Autodesk Fusion 360 part; units mm, degrees
(part 4 of 6)
  spline S54 degree 5 poles (54.1906, -36.7461) (54.1649, -36.7627) (54.114, -36.7965) (54.0391, -36.8491) (53.9417, -36.9229) (53.8236, -37.0198) (53.708, -37.1203) (53.594, -37.2229) (53.4808, -37.3266) (53.3682, -37.4312) (53.2562, -37.5365) (53.145, -37.6429) (53.0349, -37.7507) (52.9261, -37.8602) (52.8187, -37.9713) (52.7124, -38.0839) (52.6071, -38.1978) (52.5028, -38.3128) (52.3992, -38.4286) (52.2963, -38.5454) (52.1942, -38.6629) (52.0928, -38.7814) (51.9923, -38.9009) (51.8926, -39.0213) (51.7938, -39.1427) (51.6958, -39.265) (51.5985, -39.3882) (51.502, -39.5122) (51.4062, -39.637) (51.3111, -39.7625) (51.2167, -39.8889) (51.123, -40.0159) (51.03, -40.1437) (50.9377, -40.2723) (50.8462, -40.4016) (50.7553, -40.5316) (50.6651, -40.6624) (50.5755, -40.7938) (50.4867, -40.9259) (50.3985, -41.0586) (50.3109, -41.192) (50.224, -41.3261) (50.1377, -41.4608) (50.0521, -41.5961) (49.9671, -41.7321) (49.8828, -41.8686) (49.7991, -42.0058) (49.716, -42.1435) (49.6335, -42.2819) (49.5517, -42.4208) (49.4705, -42.5603) (49.3899, -42.7004) (49.3099, -42.841) (49.2305, -42.9822) (49.1517, -43.124) (49.0736, -43.2662) (48.996, -43.4091) (48.919, -43.5524) (48.8427, -43.6963) (48.7669, -43.8407) (48.6917, -43.9856) (48.6171, -44.131) (48.5431, -44.2769) (48.4697, -44.4233) (48.3969, -44.5702) (48.3246, -44.7176) (48.253, -44.8654) (48.1819, -45.0138) (48.1114, -45.1626) (48.0414, -45.3118) (47.9721, -45.4616) (47.9171, -45.5817) (47.876, -45.6721) (47.8488, -45.7324) (47.8352, -45.7626) knots 0 0 0 0 0 0 0.01428571 0.02857143 0.04285714 0.05714286 0.07142857 0.08571429 0.1 0.11428571 0.12857143 0.14285714 0.15714286 0.17142857 0.18571429 0.2 0.21428571 0.22857143 0.24285714 0.25714286 0.27142857 0.28571429 0.3 0.31428571 0.32857143 0.34285714 0.35714286 0.37142857 0.38571429 0.4 0.41428571 0.42857143 0.44285714 0.45714286 0.47142857 0.48571429 0.5 0.51428571 0.52857143 0.54285714 0.55714286 0.57142857 0.58571429 0.6 0.61428571 0.62857143 0.64285714 0.65714286 0.67142857 0.68571429 0.7 0.71428571 0.72857143 0.74285714 0.75714286 0.77142857 0.78571429 0.8 0.81428571 0.82857143 0.84285714 0.85714286 0.87142857 0.88571429 0.9 0.91428571 0.92857143 0.94285714 0.95714286 0.97142857 0.98571429 1 1 1 1 1 1
  arc A111 (47.8352, -45.7626) -> (50.4485, -49.1682) centre (111, 0) ccw
  spline S55 degree 5 poles (50.4485, -49.1682) (50.4812, -49.1629) (50.5465, -49.1523) (50.6443, -49.136) (50.7747, -49.114) (50.9372, -49.0857) (51.0995, -49.0568) (51.2615, -49.0272) (51.4232, -48.997) (51.5846, -48.966) (51.7456, -48.9344) (51.9064, -48.902) (52.0668, -48.869) (52.2269, -48.8353) (52.3866, -48.8009) (52.5461, -48.7658) (52.7051, -48.73) (52.8639, -48.6934) (53.0222, -48.6562) (53.1803, -48.6182) (53.3379, -48.5795) (53.4952, -48.5401) (53.6522, -48.5) (53.8087, -48.4591) (53.9649, -48.4175) (54.1206, -48.3752) (54.276, -48.3321) (54.431, -48.2883) (54.5856, -48.2437) (54.7397, -48.1983) (54.8935, -48.1522) (55.0468, -48.1053) (55.1996, -48.0576) (55.3521, -48.0091) (55.504, -47.9599) (55.6556, -47.9098) (55.8066, -47.859) (55.9572, -47.8073) (56.1073, -47.7549) (56.257, -47.7016) (56.4061, -47.6474) (56.5547, -47.5924) (56.7028, -47.5366) (56.8503, -47.4799) (56.9973, -47.4222) (57.1437, -47.3638) (57.2896, -47.3044) (57.4349, -47.2442) (57.5797, -47.183) (57.7238, -47.121) (57.8674, -47.0579) (58.0102, -46.9939) (58.1523, -46.9288) (58.2937, -46.8626) (58.4344, -46.7954) (58.5744, -46.7271) (58.7138, -46.658) (58.8525, -46.5879) (58.9906, -46.5169) (59.1278, -46.4447) (59.2641, -46.3712) (59.3992, -46.2961) (59.5331, -46.2194) (59.6658, -46.141) (59.7973, -46.0611) (59.928, -45.9802) (60.0582, -45.8985) (60.1877, -45.816) (60.3163, -45.7324) (60.4433, -45.6467) (60.5675, -45.5577) (60.6639, -45.4828) (60.7341, -45.424) (60.7799, -45.3836) (60.8026, -45.3631) knots -1 -1 -1 -1 -1 -1 -0.98571429 -0.97142857 -0.95714286 -0.94285714 -0.92857143 -0.91428571 -0.9 -0.88571429 -0.87142857 -0.85714286 -0.84285714 -0.82857143 -0.81428571 -0.8 -0.78571429 -0.77142857 -0.75714286 -0.74285714 -0.72857143 -0.71428571 -0.7 -0.68571429 -0.67142857 -0.65714286 -0.64285714 -0.62857143 -0.61428571 -0.6 -0.58571429 -0.57142857 -0.55714286 -0.54285714 -0.52857143 -0.51428571 -0.5 -0.48571429 -0.47142857 -0.45714286 -0.44285714 -0.42857143 -0.41428571 -0.4 -0.38571429 -0.37142857 -0.35714286 -0.34285714 -0.32857143 -0.31428571 -0.3 -0.28571429 -0.27142857 -0.25714286 -0.24285714 -0.22857143 -0.21428571 -0.2 -0.18571429 -0.17142857 -0.15714286 -0.14285714 -0.12857143 -0.11428571 -0.1 -0.08571429 -0.07142857 -0.05714286 -0.04285714 -0.02857143 -0.01428571 0 0 0 0 0 0
  line L55 (60.8026, -45.3631) -> (61.2698, -44.9409)
  arc A112 (64.054, -45.0401) -> (61.2698, -44.9409) centre (62.6108, -46.4248) ccw
  arc A113 (64.054, -45.0401) -> (65.9599, -46.946) centre (111, 0) ccw
  arc A114 (66.0591, -49.7302) -> (65.9599, -46.946) centre (64.5752, -48.3892) ccw
  line L56 (66.0591, -49.7302) -> (65.6369, -50.1974)
  spline S56 degree 5 poles (65.6369, -50.1974) (65.6164, -50.2201) (65.576, -50.2659) (65.5172, -50.3361) (65.4423, -50.4325) (65.3533, -50.5567) (65.2676, -50.6837) (65.184, -50.8123) (65.1015, -50.9418) (65.0198, -51.072) (64.9389, -51.2027) (64.859, -51.3342) (64.7806, -51.4669) (64.7039, -51.6008) (64.6288, -51.7359) (64.5553, -51.8722) (64.4831, -52.0094) (64.4121, -52.1475) (64.342, -52.2862) (64.2729, -52.4256) (64.2046, -52.5656) (64.1374, -52.7063) (64.0712, -52.8477) (64.0061, -52.9898) (63.9421, -53.1326) (63.879, -53.2762) (63.817, -53.4203) (63.7558, -53.5651) (63.6956, -53.7104) (63.6362, -53.8563) (63.5778, -54.0027) (63.5201, -54.1497) (63.4634, -54.2972) (63.4076, -54.4453) (63.3526, -54.5939) (63.2984, -54.743) (63.2451, -54.8927) (63.1927, -55.0428) (63.141, -55.1934) (63.0902, -55.3444) (63.0401, -55.496) (62.9909, -55.6479) (62.9424, -55.8004) (62.8947, -55.9532) (62.8478, -56.1065) (62.8017, -56.2603) (62.7563, -56.4144) (62.7117, -56.569) (62.6679, -56.724) (62.6248, -56.8794) (62.5825, -57.0351) (62.5409, -57.1913) (62.5, -57.3478) (62.4599, -57.5048) (62.4205, -57.6621) (62.3818, -57.8197) (62.3438, -57.9778) (62.3066, -58.1361) (62.27, -58.2949) (62.2342, -58.4539) (62.1991, -58.6134) (62.1647, -58.7731) (62.131, -58.9332) (62.098, -59.0936) (62.0656, -59.2544) (62.034, -59.4154) (62.003, -59.5768) (61.9728, -59.7385) (61.9432, -59.9005) (61.9143, -60.0628) (61.886, -60.2253) (61.864, -60.3557) (61.8477, -60.4535) (61.8371, -60.5188) (61.8318, -60.5515) knots 0 0 0 0 0 0 0.01428571 0.02857143 0.04285714 0.05714286 0.07142857 0.08571429 0.1 0.11428571 0.12857143 0.14285714 0.15714286 0.17142857 0.18571429 0.2 0.21428571 0.22857143 0.24285714 0.25714286 0.27142857 0.28571429 0.3 0.31428571 0.32857143 0.34285714 0.35714286 0.37142857 0.38571429 0.4 0.41428571 0.42857143 0.44285714 0.45714286 0.47142857 0.48571429 0.5 0.51428571 0.52857143 0.54285714 0.55714286 0.57142857 0.58571429 0.6 0.61428571 0.62857143 0.64285714 0.65714286 0.67142857 0.68571429 0.7 0.71428571 0.72857143 0.74285714 0.75714286 0.77142857 0.78571429 0.8 0.81428571 0.82857143 0.84285714 0.85714286 0.87142857 0.88571429 0.9 0.91428571 0.92857143 0.94285714 0.95714286 0.97142857 0.98571429 1 1 1 1 1 1
  arc A115 (61.8318, -60.5515) -> (65.2374, -63.1648) centre (111, 0) ccw
  spline S57 degree 5 poles (65.2374, -63.1648) (65.2676, -63.1512) (65.3279, -63.124) (65.4183, -63.0829) (65.5384, -63.0279) (65.6882, -62.9586) (65.8374, -62.8886) (65.9862, -62.8181) (66.1346, -62.747) (66.2824, -62.6754) (66.4298, -62.6031) (66.5767, -62.5303) (66.7231, -62.4569) (66.869, -62.3829) (67.0144, -62.3083) (67.1593, -62.2331) (67.3037, -62.1573) (67.4476, -62.081) (67.5909, -62.004) (67.7338, -61.9264) (67.876, -61.8483) (68.0178, -61.7695) (68.159, -61.6901) (68.2996, -61.6101) (68.4397, -61.5295) (68.5792, -61.4483) (68.7181, -61.3665) (68.8565, -61.284) (68.9942, -61.2009) (69.1314, -61.1172) (69.2679, -61.0329) (69.4039, -60.9479) (69.5392, -60.8623) (69.6739, -60.776) (69.808, -60.6891) (69.9414, -60.6015) (70.0741, -60.5133) (70.2062, -60.4245) (70.3376, -60.3349) (70.4684, -60.2447) (70.5984, -60.1538) (70.7277, -60.0623) (70.8563, -59.97) (70.9841, -59.877) (71.1111, -59.7833) (71.2375, -59.6889) (71.363, -59.5938) (71.4878, -59.498) (71.6118, -59.4015) (71.735, -59.3042) (71.8573, -59.2062) (71.9787, -59.1074) (72.0991, -59.0077) (72.2186, -58.9072) (72.3371, -58.8058) (72.4546, -58.7037) (72.5714, -58.6008) (72.6872, -58.4972) (72.8022, -58.3929) (72.9161, -58.2876) (73.0287, -58.1813) (73.1398, -58.0739) (73.2493, -57.9651) (73.3571, -57.855) (73.4635, -57.7438) (73.5688, -57.6318) (73.6734, -57.5192) (73.7771, -57.406) (73.8797, -57.292) (73.9802, -57.1764) (74.0771, -57.0583) (74.1509, -56.9609) (74.2035, -56.886) (74.2373, -56.8351) (74.2539, -56.8094) knots -1 -1 -1 -1 -1 -1 -0.98571429 -0.97142857 -0.95714286 -0.94285714 -0.92857143 -0.91428571 -0.9 -0.88571429 -0.87142857 -0.85714286 -0.84285714 -0.82857143 -0.81428571 -0.8 -0.78571429 -0.77142857 -0.75714286 -0.74285714 -0.72857143 -0.71428571 -0.7 -0.68571429 -0.67142857 -0.65714286 -0.64285714 -0.62857143 -0.61428571 -0.6 -0.58571429 -0.57142857 -0.55714286 -0.54285714 -0.52857143 -0.51428571 -0.5 -0.48571429 -0.47142857 -0.45714286 -0.44285714 -0.42857143 -0.41428571 -0.4 -0.38571429 -0.37142857 -0.35714286 -0.34285714 -0.32857143 -0.31428571 -0.3 -0.28571429 -0.27142857 -0.25714286 -0.24285714 -0.22857143 -0.21428571 -0.2 -0.18571429 -0.17142857 -0.15714286 -0.14285714 -0.12857143 -0.11428571 -0.1 -0.08571429 -0.07142857 -0.05714286 -0.04285714 -0.02857143 -0.01428571 0 0 0 0 0 0
  line L57 (74.2539, -56.8094) -> (74.5959, -56.2807)
  arc A116 (77.3109, -55.656) -> (74.5959, -56.2807) centre (76.2752, -57.3669) ccw
  arc A117 (77.3109, -55.656) -> (79.6451, -57.0036) centre (111, 0) ccw
  arc A118 (80.4615, -59.6672) -> (79.6451, -57.0036) centre (78.6812, -58.756) ccw
  line L58 (80.4615, -59.6672) -> (80.1746, -60.2278)
  spline S58 degree 5 poles (80.1746, -60.2278) (80.1607, -60.255) (80.1336, -60.3097) (80.095, -60.3928) (80.0475, -60.5053) (79.9937, -60.6483) (79.9438, -60.7931) (79.8964, -60.939) (79.8502, -61.0854) (79.8049, -61.2323) (79.7606, -61.3795) (79.7175, -61.5272) (79.6761, -61.6756) (79.6367, -61.8248) (79.5991, -61.9748) (79.5634, -62.1255) (79.5292, -62.2767) (79.4963, -62.4284) (79.4645, -62.5806) (79.4338, -62.7331) (79.4041, -62.886) (79.3756, -63.0393) (79.3483, -63.193) (79.3222, -63.3471) (79.2973, -63.5017) (79.2735, -63.6566) (79.2509, -63.8119) (79.2293, -63.9676) (79.2087, -64.1236) (79.1892, -64.2798) (79.1706, -64.4364) (79.153, -64.5933) (79.1363, -64.7505) (79.1207, -64.908) (79.1061, -65.0657) (79.0924, -65.2238) (79.0796, -65.3821) (79.0678, -65.5407) (79.0569, -65.6995) (79.0468, -65.8586) (79.0377, -66.0179) (79.0295, -66.1775) (79.0221, -66.3372) (79.0156, -66.4972) (79.01, -66.6575) (79.0052, -66.8179) (79.0013, -66.9785) (78.9983, -67.1394) (78.996, -67.3004) (78.9946, -67.4617) (78.994, -67.6231) (78.9943, -67.7847) (78.9953, -67.9465) (78.9972, -68.1085) (78.9998, -68.2706) (79.0033, -68.4329) (79.0075, -68.5954) (79.0125, -68.758) (79.0183, -68.9208) (79.0249, -69.0837) (79.0322, -69.2468) (79.0403, -69.41) (79.0492, -69.5733) (79.0588, -69.7368) (79.0692, -69.9005) (79.0803, -70.0642) (79.0922, -70.2281) (79.1048, -70.3921) (79.1181, -70.5563) (79.1322, -70.7205) (79.147, -70.8848) (79.1594, -71.0164) (79.1691, -71.1152) (79.1757, -71.181) (79.179, -71.2139) knots 0 0 0 0 0 0 0.01428571 0.02857143 0.04285714 0.05714286 0.07142857 0.08571429 0.1 0.11428571 0.12857143 0.14285714 0.15714286 0.17142857 0.18571429 0.2 0.21428571 0.22857143 0.24285714 0.25714286 0.27142857 0.28571429 0.3 0.31428571 0.32857143 0.34285714 0.35714286 0.37142857 0.38571429 0.4 0.41428571 0.42857143 0.44285714 0.45714286 0.47142857 0.48571429 0.5 0.51428571 0.52857143 0.54285714 0.55714286 0.57142857 0.58571429 0.6 0.61428571 0.62857143 0.64285714 0.65714286 0.67142857 0.68571429 0.7 0.71428571 0.72857143 0.74285714 0.75714286 0.77142857 0.78571429 0.8 0.81428571 0.82857143 0.84285714 0.85714286 0.87142857 0.88571429 0.9 0.91428571 0.92857143 0.94285714 0.95714286 0.97142857 0.98571429 1 1 1 1 1 1
  arc A119 (79.179, -71.2139) -> (83.145, -72.8567) centre (111, 0) ccw
  spline S59 degree 5 poles (83.145, -72.8567) (83.1706, -72.8358) (83.2218, -72.7939) (83.2985, -72.7309) (83.4003, -72.6466) (83.527, -72.5409) (83.6531, -72.4347) (83.7786, -72.3281) (83.9035, -72.221) (84.0277, -72.1135) (84.1514, -72.0056) (84.2744, -71.8972) (84.3969, -71.7884) (84.5186, -71.6792) (84.6398, -71.5695) (84.7603, -71.4594) (84.8801, -71.3488) (84.9993, -71.2378) (85.1179, -71.1264) (85.2358, -71.0145) (85.353, -70.9021) (85.4695, -70.7894) (85.5853, -70.6762) (85.7004, -70.5625) (85.8149, -70.4484) (85.9286, -70.3338) (86.0416, -70.2188) (86.1539, -70.1034) (86.2655, -69.9875) (86.3763, -69.8711) (86.4864, -69.7543) (86.5957, -69.637) (86.7043, -69.5193) (86.8121, -69.4011) (86.919, -69.2825) (87.0252, -69.1634) (87.1306, -69.0438) (87.2352, -68.9238) (87.339, -68.8033) (87.4419, -68.6823) (87.544, -68.5608) (87.6452, -68.4389) (87.7455, -68.3165) (87.8449, -68.1936) (87.9434, -68.0702) (88.041, -67.9464) (88.1376, -67.822) (88.2334, -67.6972) (88.3282, -67.5719) (88.422, -67.446) (88.5147, -67.3197) (88.6064, -67.1928) (88.6969, -67.0653) (88.7863, -66.9373) (88.8745, -66.8088) (88.9617, -66.6797) (89.0478, -66.5501) (89.1329, -66.4201) (89.2169, -66.2895) (89.2997, -66.1584) (89.381, -66.0266) (89.4605, -65.894) (89.5381, -65.7606) (89.6137, -65.6264) (89.6877, -65.4914) (89.7605, -65.356) (89.8323, -65.2202) (89.9032, -65.084) (89.9728, -64.9473) (90.0399, -64.8096) (90.103, -64.6704) (90.149, -64.5573) (90.1805, -64.4713) (90.2, -64.4134) (90.2094, -64.3843) knots -1 -1 -1 -1 -1 -1 -0.98571429 -0.97142857 -0.95714286 -0.94285714 -0.92857143 -0.91428571 -0.9 -0.88571429 -0.87142857 -0.85714286 -0.84285714 -0.82857143 -0.81428571 -0.8 -0.78571429 -0.77142857 -0.75714286 -0.74285714 -0.72857143 -0.71428571 -0.7 -0.68571429 -0.67142857 -0.65714286 -0.64285714 -0.62857143 -0.61428571 -0.6 -0.58571429 -0.57142857 -0.55714286 -0.54285714 -0.52857143 -0.51428571 -0.5 -0.48571429 -0.47142857 -0.45714286 -0.44285714 -0.42857143 -0.41428571 -0.4 -0.38571429 -0.37142857 -0.35714286 -0.34285714 -0.32857143 -0.31428571 -0.3 -0.28571429 -0.27142857 -0.25714286 -0.24285714 -0.22857143 -0.21428571 -0.2 -0.18571429 -0.17142857 -0.15714286 -0.14285714 -0.12857143 -0.11428571 -0.1 -0.08571429 -0.07142857 -0.05714286 -0.04285714 -0.02857143 -0.01428571 0 0 0 0 0 0
  line L59 (90.2094, -64.3843) -> (90.4029, -63.7851)
  arc A120 (92.8636, -62.4789) -> (90.4029, -63.7851) centre (92.3061, -64.3996) ccw
  arc A121 (92.8636, -62.4789) -> (95.4671, -63.1765) centre (111, 0) ccw
  arc A122 (96.9451, -65.538) -> (95.4671, -63.1765) centre (94.9896, -65.1187) ccw
  line L60 (96.9451, -65.538) -> (96.8131, -66.1537)
  spline S60 degree 5 poles (96.8131, -66.1537) (96.8067, -66.1836) (96.7946, -66.2435) (96.7788, -66.3338) (96.7621, -66.4547) (96.7471, -66.6068) (96.7364, -66.7596) (96.7284, -66.9128) (96.7217, -67.0662) (96.716, -67.2197) (96.7113, -67.3734) (96.7079, -67.5272) (96.7063, -67.6813) (96.7068, -67.8356) (96.7093, -67.9902) (96.7138, -68.145) (96.7199, -68.2999) (96.7274, -68.455) (96.7361, -68.6102) (96.7459, -68.7655) (96.7568, -68.9208) (96.769, -69.0763) (96.7823, -69.2318) (96.797, -69.3875) (96.813, -69.5432) (96.8301, -69.699) (96.8485, -69.8549) (96.8679, -70.0108) (96.8884, -70.1668) (96.9099, -70.3228) (96.9325, -70.4789) (96.9561, -70.635) (96.9807, -70.7911) (97.0064, -70.9473) (97.0331, -71.1034) (97.0607, -71.2596) (97.0894, -71.4159) (97.119, -71.5721) (97.1496, -71.7284) (97.1811, -71.8846) (97.2135, -72.0409) (97.2468, -72.1971) (97.2811, -72.3533) (97.3162, -72.5096) (97.3523, -72.6658) (97.3892, -72.822) (97.427, -72.9782) (97.4656, -73.1343) (97.5052, -73.2905) (97.5455, -73.4466) (97.5868, -73.6026) (97.6288, -73.7587) (97.6717, -73.9147) (97.7154, -74.0707) (97.7599, -74.2266) (97.8053, -74.3825) (97.8514, -74.5383) (97.8983, -74.6941) (97.9461, -74.8498) (97.9946, -75.0055) (98.0439, -75.1611) (98.0939, -75.3167) (98.1448, -75.4722) (98.1964, -75.6276) (98.2488, -75.783) (98.3019, -75.9383) (98.3558, -76.0935) (98.4104, -76.2487) (98.4658, -76.4037) (98.5219, -76.5587) (98.5787, -76.7137) (98.6248, -76.8375) (98.6597, -76.9304) (98.6831, -76.9923) (98.6948, -77.0233) knots 0 0 0 0 0 0 0.01428571 0.02857143 0.04285714 0.05714286 0.07142857 0.08571429 0.1 0.11428571 0.12857143 0.14285714 0.15714286 0.17142857 0.18571429 0.2 0.21428571 0.22857143 0.24285714 0.25714286 0.27142857 0.28571429 0.3 0.31428571 0.32857143 0.34285714 0.35714286 0.37142857 0.38571429 0.4 0.41428571 0.42857143 0.44285714 0.45714286 0.47142857 0.48571429 0.5 0.51428571 0.52857143 0.54285714 0.55714286 0.57142857 0.58571429 0.6 0.61428571 0.62857143 0.64285714 0.65714286 0.67142857 0.68571429 0.7 0.71428571 0.72857143 0.74285714 0.75714286 0.77142857 0.78571429 0.8 0.81428571 0.82857143 0.84285714 0.85714286 0.87142857 0.88571429 0.9 0.91428571 0.92857143 0.94285714 0.95714286 0.97142857 0.98571429 1 1 1 1 1 1
  arc A123 (98.6948, -77.0233) -> (102.9508, -77.5836) centre (111, 0) ccw
  spline S61 degree 5 poles (102.9508, -77.5836) (102.9702, -77.5567) (103.0088, -77.503) (103.0665, -77.4223) (103.1431, -77.3146) (103.2381, -77.1796) (103.3324, -77.0444) (103.426, -76.909) (103.5189, -76.7732) (103.6111, -76.6373) (103.7027, -76.501) (103.7935, -76.3645) (103.8835, -76.2277) (103.9729, -76.0906) (104.0615, -75.9533) (104.1494, -75.8158) (104.2366, -75.678) (104.323, -75.5399) (104.4087, -75.4016) (104.4935, -75.263) (104.5777, -75.1242) (104.661, -74.9851) (104.7436, -74.8457) (104.8254, -74.7061) (104.9064, -74.5663) (104.9866, -74.4262) (105.066, -74.2859) (105.1446, -74.1453) (105.2224, -74.0045) (105.2993, -73.8634) (105.3754, -73.7221) (105.4507, -73.5805) (105.5251, -73.4387) (105.5986, -73.2966) (105.6712, -73.1543) (105.743, -73.0118) (105.8138, -72.869) (105.8838, -72.726) (105.9528, -72.5828) (106.0209, -72.4393) (106.0881, -72.2956) (106.1543, -72.1516) (106.2195, -72.0074) (106.2837, -71.863) (106.3469, -71.7183) (106.4091, -71.5734) (106.4703, -71.4283) (106.5304, -71.2829) (106.5896, -71.1373) (106.6476, -70.9915) (106.7045, -70.8454) (106.7602, -70.6991) (106.8147, -70.5526) (106.8679, -70.4058) (106.9198, -70.2588) (106.9706, -70.1116) (107.0202, -69.9641) (107.0688, -69.8165) (107.1162, -69.6686) (107.1622, -69.5205) (107.2066, -69.3722) (107.249, -69.2235) (107.2894, -69.0746) (107.3278, -68.9254) (107.3644, -68.7759) (107.3996, -68.6262) (107.4338, -68.4764) (107.467, -68.3265) (107.4989, -68.1765) (107.5281, -68.0261) (107.553, -67.8753) (107.5682, -67.7542) (107.5763, -67.663) (107.5801, -67.602) (107.5817, -67.5715) knots -1 -1 -1 -1 -1 -1 -0.98571429 -0.97142857 -0.95714286 -0.94285714 -0.92857143 -0.91428571 -0.9 -0.88571429 -0.87142857 -0.85714286 -0.84285714 -0.82857143 -0.81428571 -0.8 -0.78571429 -0.77142857 -0.75714286 -0.74285714 -0.72857143 -0.71428571 -0.7 -0.68571429 -0.67142857 -0.65714286 -0.64285714 -0.62857143 -0.61428571 -0.6 -0.58571429 -0.57142857 -0.55714286 -0.54285714 -0.52857143 -0.51428571 -0.5 -0.48571429 -0.47142857 -0.45714286 -0.44285714 -0.42857143 -0.41428571 -0.4 -0.38571429 -0.37142857 -0.35714286 -0.34285714 -0.32857143 -0.31428571 -0.3 -0.28571429 -0.27142857 -0.25714286 -0.24285714 -0.22857143 -0.21428571 -0.2 -0.18571429 -0.17142857 -0.15714286 -0.14285714 -0.12857143 -0.11428571 -0.1 -0.08571429 -0.07142857 -0.05714286 -0.04285714 -0.02857143 -0.01428571 0 0 0 0 0 0
  line L61 (107.5817, -67.5715) -> (107.6135, -66.9426)
  arc A124 (109.6523, -65.044) -> (107.6135, -66.9426) centre (109.6109, -67.0436) ccw
  arc A125 (109.6523, -65.044) -> (112.3477, -65.044) centre (111, 0) ccw
  arc A126 (114.3865, -66.9426) -> (112.3477, -65.044) centre (112.3891, -67.0436) ccw
  line L62 (114.3865, -66.9426) -> (114.4183, -67.5715)
  spline S62 degree 5 poles (114.4183, -67.5715) (114.4199, -67.602) (114.4237, -67.663) (114.4318, -67.7542) (114.447, -67.8753) (114.4719, -68.0261) (114.5011, -68.1765) (114.533, -68.3265) (114.5662, -68.4764) (114.6004, -68.6262) (114.6356, -68.7759) (114.6722, -68.9254) (114.7106, -69.0746) (114.751, -69.2235) (114.7934, -69.3722) (114.8378, -69.5205) (114.8838, -69.6686) (114.9312, -69.8165) (114.9798, -69.9641) (115.0294, -70.1116) (115.0802, -70.2588) (115.1321, -70.4058) (115.1853, -70.5526) (115.2398, -70.6991) (115.2955, -70.8454) (115.3524, -70.9915) (115.4104, -71.1373) (115.4696, -71.2829) (115.5297, -71.4283) (115.5909, -71.5734) (115.6531, -71.7183) (115.7163, -71.863) (115.7805, -72.0074) (115.8457, -72.1516) (115.9119, -72.2956) (115.9791, -72.4393) (116.0472, -72.5828) (116.1162, -72.726) (116.1862, -72.869) (116.257, -73.0118) (116.3288, -73.1543) (116.4014, -73.2966) (116.4749, -73.4387) (116.5493, -73.5805) (116.6246, -73.7221) (116.7007, -73.8634) (116.7776, -74.0045) (116.8554, -74.1453) (116.934, -74.2859) (117.0134, -74.4262) (117.0936, -74.5663) (117.1746, -74.7061) (117.2564, -74.8457) (117.339, -74.9851) (117.4223, -75.1242) (117.5065, -75.263) (117.5913, -75.4016) (117.677, -75.5399) (117.7634, -75.678) (117.8506, -75.8158) (117.9385, -75.9533) (118.0271, -76.0906) (118.1165, -76.2277) (118.2065, -76.3645) (118.2973, -76.501) (118.3889, -76.6373) (118.4811, -76.7732) (118.574, -76.909) (118.6676, -77.0444) (118.7619, -77.1796) (118.8569, -77.3146) (118.9335, -77.4223) (118.9912, -77.503) (119.0298, -77.5567) (119.0492, -77.5836) knots 0 0 0 0 0 0 0.01428571 0.02857143 0.04285714 0.05714286 0.07142857 0.08571429 0.1 0.11428571 0.12857143 0.14285714 0.15714286 0.17142857 0.18571429 0.2 0.21428571 0.22857143 0.24285714 0.25714286 0.27142857 0.28571429 0.3 0.31428571 0.32857143 0.34285714 0.35714286 0.37142857 0.38571429 0.4 0.41428571 0.42857143 0.44285714 0.45714286 0.47142857 0.48571429 0.5 0.51428571 0.52857143 0.54285714 0.55714286 0.57142857 0.58571429 0.6 0.61428571 0.62857143 0.64285714 0.65714286 0.67142857 0.68571429 0.7 0.71428571 0.72857143 0.74285714 0.75714286 0.77142857 0.78571429 0.8 0.81428571 0.82857143 0.84285714 0.85714286 0.87142857 0.88571429 0.9 0.91428571 0.92857143 0.94285714 0.95714286 0.97142857 0.98571429 1 1 1 1 1 1
  arc A127 (119.0492, -77.5836) -> (123.3052, -77.0233) centre (111, 0) ccw
  spline S63 degree 5 poles (123.3052, -77.0233) (123.3169, -76.9923) (123.3403, -76.9304) (123.3752, -76.8375) (123.4213, -76.7137) (123.4781, -76.5587) (123.5342, -76.4037) (123.5896, -76.2487) (123.6442, -76.0935) (123.6981, -75.9383) (123.7512, -75.783) (123.8036, -75.6276) (123.8552, -75.4722) (123.9061, -75.3167) (123.9561, -75.1611) (124.0054, -75.0055) (124.0539, -74.8498) (124.1017, -74.6941) (124.1486, -74.5383) (124.1947, -74.3825) (124.2401, -74.2266) (124.2846, -74.0707) (124.3283, -73.9147) (124.3712, -73.7587) (124.4132, -73.6026) (124.4545, -73.4466) (124.4948, -73.2905) (124.5344, -73.1343) (124.573, -72.9782) (124.6108, -72.822) (124.6477, -72.6658) (124.6838, -72.5096) (124.7189, -72.3533) (124.7532, -72.1971) (124.7865, -72.0409) (124.8189, -71.8846) (124.8504, -71.7284) (124.881, -71.5721) (124.9106, -71.4159) (124.9393, -71.2596) (124.9669, -71.1034) (124.9936, -70.9473) (125.0193, -70.7911) (125.0439, -70.635) (125.0675, -70.4789) (125.0901, -70.3228) (125.1116, -70.1668) (125.1321, -70.0108) (125.1515, -69.8549) (125.1699, -69.699) (125.187, -69.5432) (125.203, -69.3875) (125.2177, -69.2318) (125.231, -69.0763) (125.2432, -68.9208) (125.2541, -68.7655) (125.2639, -68.6102) (125.2726, -68.455) (125.2801, -68.2999) (125.2862, -68.145) (125.2907, -67.9902) (125.2932, -67.8356) (125.2937, -67.6813) (125.2921, -67.5272) (125.2887, -67.3734) (125.284, -67.2197) (125.2783, -67.0662) (125.2716, -66.9128) (125.2636, -66.7596) (125.2529, -66.6068) (125.2379, -66.4547) (125.2212, -66.3338) (125.2054, -66.2435) (125.1933, -66.1836) (125.1869, -66.1537) knots -1 -1 -1 -1 -1 -1 -0.98571429 -0.97142857 -0.95714286 -0.94285714 -0.92857143 -0.91428571 -0.9 -0.88571429 -0.87142857 -0.85714286 -0.84285714 -0.82857143 -0.81428571 -0.8 -0.78571429 -0.77142857 -0.75714286 -0.74285714 -0.72857143 -0.71428571 -0.7 -0.68571429 -0.67142857 -0.65714286 -0.64285714 -0.62857143 -0.61428571 -0.6 -0.58571429 -0.57142857 -0.55714286 -0.54285714 -0.52857143 -0.51428571 -0.5 -0.48571429 -0.47142857 -0.45714286 -0.44285714 -0.42857143 -0.41428571 -0.4 -0.38571429 -0.37142857 -0.35714286 -0.34285714 -0.32857143 -0.31428571 -0.3 -0.28571429 -0.27142857 -0.25714286 -0.24285714 -0.22857143 -0.21428571 -0.2 -0.18571429 -0.17142857 -0.15714286 -0.14285714 -0.12857143 -0.11428571 -0.1 -0.08571429 -0.07142857 -0.05714286 -0.04285714 -0.02857143 -0.01428571 0 0 0 0 0 0
  line L63 (125.1869, -66.1537) -> (125.0549, -65.538)
  arc A128 (126.5329, -63.1765) -> (125.0549, -65.538) centre (127.0104, -65.1187) ccw
  arc A129 (126.5329, -63.1765) -> (129.1364, -62.4789) centre (111, 0) ccw
  arc A130 (131.5971, -63.7851) -> (129.1364, -62.4789) centre (129.6939, -64.3996) ccw
  line L64 (131.5971, -63.7851) -> (131.7906, -64.3843)
  spline S64 degree 5 poles (131.7906, -64.3843) (131.8, -64.4134) (131.8195, -64.4713) (131.851, -64.5573) (131.897, -64.6704) (131.9601, -64.8096) (132.0272, -64.9473) (132.0968, -65.084) (132.1677, -65.2202) (132.2395, -65.356) (132.3123, -65.4914) (132.3863, -65.6264) (132.4619, -65.7606) (132.5395, -65.894) (132.619, -66.0266) (132.7003, -66.1584) (132.7831, -66.2895) (132.8671, -66.4201) (132.9522, -66.5501) (133.0383, -66.6797) (133.1255, -66.8088) (133.2137, -66.9373) (133.3031, -67.0653) (133.3936, -67.1928) (133.4853, -67.3197) (133.578, -67.446) (133.6718, -67.5719) (133.7666, -67.6972) (133.8624, -67.822) (133.959, -67.9464) (134.0566, -68.0702) (134.1551, -68.1936) (134.2545, -68.3165) (134.3548, -68.4389) (134.456, -68.5608) (134.5581, -68.6823) (134.661, -68.8033) (134.7648, -68.9238) (134.8694, -69.0438) (134.9748, -69.1634) (135.081, -69.2825) (135.1879, -69.4011) (135.2957, -69.5193) (135.4043, -69.637) (135.5136, -69.7543) (135.6237, -69.8711) (135.7345, -69.9875) (135.8461, -70.1034) (135.9584, -70.2188) (136.0714, -70.3338) (136.1851, -70.4484) (136.2996, -70.5625) (136.4147, -70.6762) (136.5305, -70.7894) (136.647, -70.9021) (136.7642, -71.0145) (136.8821, -71.1264) (137.0007, -71.2378) (137.1199, -71.3488) (137.2397, -71.4594) (137.3602, -71.5695) (137.4814, -71.6792) (137.6031, -71.7884) (137.7256, -71.8972) (137.8486, -72.0056) (137.9723, -72.1135) (138.0965, -72.221) (138.2214, -72.3281) (138.3469, -72.4347) (138.473, -72.5409) (138.5997, -72.6466) (138.7015, -72.7309) (138.7782, -72.7939) (138.8294, -72.8358) (138.855, -72.8567) knots 0 0 0 0 0 0 0.01428571 0.02857143 0.04285714 0.05714286 0.07142857 0.08571429 0.1 0.11428571 0.12857143 0.14285714 0.15714286 0.17142857 0.18571429 0.2 0.21428571 0.22857143 0.24285714 0.25714286 0.27142857 0.28571429 0.3 0.31428571 0.32857143 0.34285714 0.35714286 0.37142857 0.38571429 0.4 0.41428571 0.42857143 0.44285714 0.45714286 0.47142857 0.48571429 0.5 0.51428571 0.52857143 0.54285714 0.55714286 0.57142857 0.58571429 0.6 0.61428571 0.62857143 0.64285714 0.65714286 0.67142857 0.68571429 0.7 0.71428571 0.72857143 0.74285714 0.75714286 0.77142857 0.78571429 0.8 0.81428571 0.82857143 0.84285714 0.85714286 0.87142857 0.88571429 0.9 0.91428571 0.92857143 0.94285714 0.95714286 0.97142857 0.98571429 1 1 1 1 1 1
  arc A131 (138.855, -72.8567) -> (142.821, -71.2139) centre (111, 0) ccw
  spline S65 degree 5 poles (142.821, -71.2139) (142.8243, -71.181) (142.8309, -71.1152) (142.8406, -71.0164) (142.853, -70.8848) (142.8678, -70.7205) (142.8819, -70.5563) (142.8952, -70.3921) (142.9078, -70.2281) (142.9197, -70.0642) (142.9308, -69.9005) (142.9412, -69.7368) (142.9508, -69.5733) (142.9597, -69.41) (142.9678, -69.2468) (142.9751, -69.0837) (142.9817, -68.9208) (142.9875, -68.758) (142.9925, -68.5954) (142.9967, -68.4329) (143.0002, -68.2706) (143.0028, -68.1085) (143.0047, -67.9465) (143.0057, -67.7847) (143.006, -67.6231) (143.0054, -67.4617) (143.004, -67.3004) (143.0017, -67.1394) (142.9987, -66.9785) (142.9948, -66.8179) (142.99, -66.6575) (142.9844, -66.4972) (142.9779, -66.3372) (142.9705, -66.1775) (142.9623, -66.0179) (142.9532, -65.8586) (142.9431, -65.6995) (142.9322, -65.5407) (142.9204, -65.3821) (142.9076, -65.2238) (142.8939, -65.0657) (142.8793, -64.908) (142.8637, -64.7505) (142.847, -64.5933) (142.8294, -64.4364) (142.8108, -64.2798) (142.7913, -64.1236) (142.7707, -63.9676) (142.7491, -63.8119) (142.7265, -63.6566) (142.7027, -63.5017) (142.6778, -63.3471) (142.6517, -63.193) (142.6244, -63.0393) (142.5959, -62.886) (142.5662, -62.7331) (142.5355, -62.5806) (142.5037, -62.4284) (142.4708, -62.2767) (142.4366, -62.1255) (142.4009, -61.9748) (142.3633, -61.8248) (142.3239, -61.6756) (142.2825, -61.5272) (142.2394, -61.3795) (142.1951, -61.2323) (142.1498, -61.0854) (142.1036, -60.939) (142.0562, -60.7931) (142.0063, -60.6483) (141.9525, -60.5053) (141.905, -60.3928) (141.8664, -60.3097) (141.8393, -60.255) (141.8254, -60.2278) knots -1 -1 -1 -1 -1 -1 -0.98571429 -0.97142857 -0.95714286 -0.94285714 -0.92857143 -0.91428571 -0.9 -0.88571429 -0.87142857 -0.85714286 -0.84285714 -0.82857143 -0.81428571 -0.8 -0.78571429 -0.77142857 -0.75714286 -0.74285714 -0.72857143 -0.71428571 -0.7 -0.68571429 -0.67142857 -0.65714286 -0.64285714 -0.62857143 -0.61428571 -0.6 -0.58571429 -0.57142857 -0.55714286 -0.54285714 -0.52857143 -0.51428571 -0.5 -0.48571429 -0.47142857 -0.45714286 -0.44285714 -0.42857143 -0.41428571 -0.4 -0.38571429 -0.37142857 -0.35714286 -0.34285714 -0.32857143 -0.31428571 -0.3 -0.28571429 -0.27142857 -0.25714286 -0.24285714 -0.22857143 -0.21428571 -0.2 -0.18571429 -0.17142857 -0.15714286 -0.14285714 -0.12857143 -0.11428571 -0.1 -0.08571429 -0.07142857 -0.05714286 -0.04285714 -0.02857143 -0.01428571 0 0 0 0 0 0
  line L65 (141.8254, -60.2278) -> (141.5385, -59.6672)
  arc A132 (142.3549, -57.0036) -> (141.5385, -59.6672) centre (143.3188, -58.756) ccw
  arc A133 (142.3549, -57.0036) -> (144.6891, -55.656) centre (111, 0) ccw
  arc A134 (147.4041, -56.2807) -> (144.6891, -55.656) centre (145.7248, -57.3669) ccw
  line L66 (147.4041, -56.2807) -> (147.7461, -56.8094)
  spline S66 degree 5 poles (147.7461, -56.8094) (147.7627, -56.8351) (147.7965, -56.886) (147.8491, -56.9609) (147.9229, -57.0583) (148.0198, -57.1764) (148.1203, -57.292) (148.2229, -57.406) (148.3266, -57.5192) (148.4312, -57.6318) (148.5365, -57.7438) (148.6429, -57.855) (148.7507, -57.9651) (148.8602, -58.0739) (148.9713, -58.1813) (149.0839, -58.2876) (149.1978, -58.3929) (149.3128, -58.4972) (149.4286, -58.6008) (149.5454, -58.7037) (149.6629, -58.8058) (149.7814, -58.9072) (149.9009, -59.0077) (150.0213, -59.1074) (150.1427, -59.2062) (150.265, -59.3042) (150.3882, -59.4015) (150.5122, -59.498) (150.637, -59.5938) (150.7625, -59.6889) (150.8889, -59.7833) (151.0159, -59.877) (151.1437, -59.97) (151.2723, -60.0623) (151.4016, -60.1538) (151.5316, -60.2447) (151.6624, -60.3349) (151.7938, -60.4245) (151.9259, -60.5133) (152.0586, -60.6015) (152.192, -60.6891) (152.3261, -60.776) (152.4608, -60.8623) (152.5961, -60.9479) (152.7321, -61.0329) (152.8686, -61.1172) (153.0058, -61.2009) (153.1435, -61.284) (153.2819, -61.3665) (153.4208, -61.4483) (153.5603, -61.5295) (153.7004, -61.6101) (153.841, -61.6901) (153.9822, -61.7695) (154.124, -61.8483) (154.2662, -61.9264) (154.4091, -62.004) (154.5524, -62.081) (154.6963, -62.1573) (154.8407, -62.2331) (154.9856, -62.3083) (155.131, -62.3829) (155.2769, -62.4569) (155.4233, -62.5303) (155.5702, -62.6031) (155.7176, -62.6754) (155.8654, -62.747) (156.0138, -62.8181) (156.1626, -62.8886) (156.3118, -62.9586) (156.4616, -63.0279) (156.5817, -63.0829) (156.6721, -63.124) (156.7324, -63.1512) (156.7626, -63.1648) knots 0 0 0 0 0 0 0.01428571 0.02857143 0.04285714 0.05714286 0.07142857 0.08571429 0.1 0.11428571 0.12857143 0.14285714 0.15714286 0.17142857 0.18571429 0.2 0.21428571 0.22857143 0.24285714 0.25714286 0.27142857 0.28571429 0.3 0.31428571 0.32857143 0.34285714 0.35714286 0.37142857 0.38571429 0.4 0.41428571 0.42857143 0.44285714 0.45714286 0.47142857 0.48571429 0.5 0.51428571 0.52857143 0.54285714 0.55714286 0.57142857 0.58571429 0.6 0.61428571 0.62857143 0.64285714 0.65714286 0.67142857 0.68571429 0.7 0.71428571 0.72857143 0.74285714 0.75714286 0.77142857 0.78571429 0.8 0.81428571 0.82857143 0.84285714 0.85714286 0.87142857 0.88571429 0.9 0.91428571 0.92857143 0.94285714 0.95714286 0.97142857 0.98571429 1 1 1 1 1 1
  arc A135 (156.7626, -63.1648) -> (160.1682, -60.5515) centre (111, 0) ccw
  spline S67 degree 5 poles (160.1682, -60.5515) (160.1629, -60.5188) (160.1523, -60.4535) (160.136, -60.3557) (160.114, -60.2253) (160.0857, -60.0628) (160.0568, -59.9005) (160.0272, -59.7385) (159.997, -59.5768) (159.966, -59.4154) (159.9344, -59.2544) (159.902, -59.0936) (159.869, -58.9332) (159.8353, -58.7731) (159.8009, -58.6134) (159.7658, -58.4539) (159.73, -58.2949) (159.6934, -58.1361) (159.6562, -57.9778) (159.6182, -57.8197) (159.5795, -57.6621) (159.5401, -57.5048) (159.5, -57.3478) (159.4591, -57.1913) (159.4175, -57.0351) (159.3752, -56.8794) (159.3321, -56.724) (159.2883, -56.569) (159.2437, -56.4144) (159.1983, -56.2603) (159.1522, -56.1065) (159.1053, -55.9532) (159.0576, -55.8004) (159.0091, -55.6479) (158.9599, -55.496) (158.9098, -55.3444) (158.859, -55.1934) (158.8073, -55.0428) (158.7549, -54.8927) (158.7016, -54.743) (158.6474, -54.5939) (158.5924, -54.4453) (158.5366, -54.2972) (158.4799, -54.1497) (158.4222, -54.0027) (158.3638, -53.8563) (158.3044, -53.7104) (158.2442, -53.5651) (158.183, -53.4203) (158.121, -53.2762) (158.0579, -53.1326) (157.9939, -52.9898) (157.9288, -52.8477) (157.8626, -52.7063) (157.7954, -52.5656) (157.7271, -52.4256) (157.658, -52.2862) (157.5879, -52.1475) (157.5169, -52.0094) (157.4447, -51.8722) (157.3712, -51.7359) (157.2961, -51.6008) (157.2194, -51.4669) (157.141, -51.3342) (157.0611, -51.2027) (156.9802, -51.072) (156.8985, -50.9418) (156.816, -50.8123) (156.7324, -50.6837) (156.6467, -50.5567) (156.5577, -50.4325) (156.4828, -50.3361) (156.424, -50.2659) (156.3836, -50.2201) (156.3631, -50.1974) knots -1 -1 -1 -1 -1 -1 -0.98571429 -0.97142857 -0.95714286 -0.94285714 -0.92857143 -0.91428571 -0.9 -0.88571429 -0.87142857 -0.85714286 -0.84285714 -0.82857143 -0.81428571 -0.8 -0.78571429 -0.77142857 -0.75714286 -0.74285714 -0.72857143 -0.71428571 -0.7 -0.68571429 -0.67142857 -0.65714286 -0.64285714 -0.62857143 -0.61428571 -0.6 -0.58571429 -0.57142857 -0.55714286 -0.54285714 -0.52857143 -0.51428571 -0.5 -0.48571429 -0.47142857 -0.45714286 -0.44285714 -0.42857143 -0.41428571 -0.4 -0.38571429 -0.37142857 -0.35714286 -0.34285714 -0.32857143 -0.31428571 -0.3 -0.28571429 -0.27142857 -0.25714286 -0.24285714 -0.22857143 -0.21428571 -0.2 -0.18571429 -0.17142857 -0.15714286 -0.14285714 -0.12857143 -0.11428571 -0.1 -0.08571429 -0.07142857 -0.05714286 -0.04285714 -0.02857143 -0.01428571 0 0 0 0 0 0
  line L67 (156.3631, -50.1974) -> (155.9409, -49.7302)
  arc A136 (156.0401, -46.946) -> (155.9409, -49.7302) centre (157.4248, -48.3892) ccw
  arc A137 (156.0401, -46.946) -> (157.946, -45.0401) centre (111, 0) ccw
  arc A138 (160.7302, -44.9409) -> (157.946, -45.0401) centre (159.3892, -46.4248) ccw
  line L68 (160.7302, -44.9409) -> (161.1974, -45.3631)
  spline S68 degree 5 poles (161.1974, -45.3631) (161.2201, -45.3836) (161.2659, -45.424) (161.3361, -45.4828) (161.4325, -45.5577) (161.5567, -45.6467) (161.6837, -45.7324) (161.8123, -45.816) (161.9418, -45.8985) (162.072, -45.9802) (162.2027, -46.0611) (162.3342, -46.141) (162.4669, -46.2194) (162.6008, -46.2961) (162.7359, -46.3712) (162.8722, -46.4447) (163.0094, -46.5169) (163.1475, -46.5879) (163.2862, -46.658) (163.4256, -46.7271) (163.5656, -46.7954) (163.7063, -46.8626) (163.8477, -46.9288) (163.9898, -46.9939) (164.1326, -47.0579) (164.2762, -47.121) (164.4203, -47.183) (164.5651, -47.2442) (164.7104, -47.3044) (164.8563, -47.3638) (165.0027, -47.4222) (165.1497, -47.4799) (165.2972, -47.5366) (165.4453, -47.5924) (165.5939, -47.6474) (165.743, -47.7016) (165.8927, -47.7549) (166.0428, -47.8073) (166.1934, -47.859) (166.3444, -47.9098) (166.496, -47.9599) (166.6479, -48.0091) (166.8004, -48.0576) (166.9532, -48.1053) (167.1065, -48.1522) (167.2603, -48.1983) (167.4144, -48.2437) (167.569, -48.2883) (167.724, -48.3321) (167.8794, -48.3752) (168.0351, -48.4175) (168.1913, -48.4591) (168.3478, -48.5) (168.5048, -48.5401) (168.6621, -48.5795) (168.8197, -48.6182) (168.9778, -48.6562) (169.1361, -48.6934) (169.2949, -48.73) (169.4539, -48.7658) (169.6134, -48.8009) (169.7731, -48.8353) (169.9332, -48.869) (170.0936, -48.902) (170.2544, -48.9344) (170.4154, -48.966) (170.5768, -48.997) (170.7385, -49.0272) (170.9005, -49.0568) (171.0628, -49.0857) (171.2253, -49.114) (171.3557, -49.136) (171.4535, -49.1523) (171.5188, -49.1629) (171.5515, -49.1682) knots 0 0 0 0 0 0 0.01428571 0.02857143 0.04285714 0.05714286 0.07142857 0.08571429 0.1 0.11428571 0.12857143 0.14285714 0.15714286 0.17142857 0.18571429 0.2 0.21428571 0.22857143 0.24285714 0.25714286 0.27142857 0.28571429 0.3 0.31428571 0.32857143 0.34285714 0.35714286 0.37142857 0.38571429 0.4 0.41428571 0.42857143 0.44285714 0.45714286 0.47142857 0.48571429 0.5 0.51428571 0.52857143 0.54285714 0.55714286 0.57142857 0.58571429 0.6 0.61428571 0.62857143 0.64285714 0.65714286 0.67142857 0.68571429 0.7 0.71428571 0.72857143 0.74285714 0.75714286 0.77142857 0.78571429 0.8 0.81428571 0.82857143 0.84285714 0.85714286 0.87142857 0.88571429 0.9 0.91428571 0.92857143 0.94285714 0.95714286 0.97142857 0.98571429 1 1 1 1 1 1
  arc A139 (171.5515, -49.1682) -> (174.1648, -45.7626) centre (111, 0) ccw
  spline S69 degree 5 poles (174.1648, -45.7626) (174.1512, -45.7324) (174.124, -45.6721) (174.0829, -45.5817) (174.0279, -45.4616) (173.9586, -45.3118) (173.8886, -45.1626) (173.8181, -45.0138) (173.747, -44.8654) (173.6754, -44.7176) (173.6031, -44.5702) (173.5303, -44.4233) (173.4569, -44.2769) (173.3829, -44.131) (173.3083, -43.9856) (173.2331, -43.8407) (173.1573, -43.6963) (173.081, -43.5524) (173.004, -43.4091) (172.9264, -43.2662) (172.8483, -43.124) (172.7695, -42.9822) (172.6901, -42.841) (172.6101, -42.7004) (172.5295, -42.5603) (172.4483, -42.4208) (172.3665, -42.2819) (172.284, -42.1435) (172.2009, -42.0058) (172.1172, -41.8686) (172.0329, -41.7321) (171.9479, -41.5961) (171.8623, -41.4608) (171.776, -41.3261) (171.6891, -41.192) (171.6015, -41.0586) (171.5133, -40.9259) (171.4245, -40.7938) (171.3349, -40.6624) (171.2447, -40.5316) (171.1538, -40.4016) (171.0623, -40.2723) (170.97, -40.1437) (170.877, -40.0159) (170.7833, -39.8889) (170.6889, -39.7625) (170.5938, -39.637) (170.498, -39.5122) (170.4015, -39.3882) (170.3042, -39.265) (170.2062, -39.1427) (170.1074, -39.0213) (170.0077, -38.9009) (169.9072, -38.7814) (169.8058, -38.6629) (169.7037, -38.5454) (169.6008, -38.4286) (169.4972, -38.3128) (169.3929, -38.1978) (169.2876, -38.0839) (169.1813, -37.9713) (169.0739, -37.8602) (168.9651, -37.7507) (168.855, -37.6429) (168.7438, -37.5365) (168.6318, -37.4312) (168.5192, -37.3266) (168.406, -37.2229) (168.292, -37.1203) (168.1764, -37.0198) (168.0583, -36.9229) (167.9609, -36.8491) (167.886, -36.7965) (167.8351, -36.7627) (167.8094, -36.7461) knots -1 -1 -1 -1 -1 -1 -0.98571429 -0.97142857 -0.95714286 -0.94285714 -0.92857143 -0.91428571 -0.9 -0.88571429 -0.87142857 -0.85714286 -0.84285714 -0.82857143 -0.81428571 -0.8 -0.78571429 -0.77142857 -0.75714286 -0.74285714 -0.72857143 -0.71428571 -0.7 -0.68571429 -0.67142857 -0.65714286 -0.64285714 -0.62857143 -0.61428571 -0.6 -0.58571429 -0.57142857 -0.55714286 -0.54285714 -0.52857143 -0.51428571 -0.5 -0.48571429 -0.47142857 -0.45714286 -0.44285714 -0.42857143 -0.41428571 -0.4 -0.38571429 -0.37142857 -0.35714286 -0.34285714 -0.32857143 -0.31428571 -0.3 -0.28571429 -0.27142857 -0.25714286 -0.24285714 -0.22857143 -0.21428571 -0.2 -0.18571429 -0.17142857 -0.15714286 -0.14285714 -0.12857143 -0.11428571 -0.1 -0.08571429 -0.07142857 -0.05714286 -0.04285714 -0.02857143 -0.01428571 0 0 0 0 0 0
  line L69 (167.8094, -36.7461) -> (167.2807, -36.4041)
  arc A140 (166.656, -33.6891) -> (167.2807, -36.4041) centre (168.3669, -34.7248) ccw
  arc A141 (166.656, -33.6891) -> (168.0036, -31.3549) centre (111, 0) ccw
  arc A142 (170.6672, -30.5385) -> (168.0036, -31.3549) centre (169.756, -32.3188) ccw
  line L70 (170.6672, -30.5385) -> (171.2278, -30.8254)
  spline S70 degree 5 poles (171.2278, -30.8254) (171.255, -30.8393) (171.3097, -30.8664) (171.3928, -30.905) (171.5053, -30.9525) (171.6483, -31.0063) (171.7931, -31.0562) (171.939, -31.1036) (172.0854, -31.1498) (172.2323, -31.1951) (172.3795, -31.2394) (172.5272, -31.2825) (172.6756, -31.3239) (172.8248, -31.3633) (172.9748, -31.4009) (173.1255, -31.4366) (173.2767, -31.4708) (173.4284, -31.5037) (173.5806, -31.5355) (173.7331, -31.5662) (173.886, -31.5959) (174.0393, -31.6244) (174.193, -31.6517) (174.3471, -31.6778) (174.5017, -31.7027) (174.6566, -31.7265) (174.8119, -31.7491) (174.9676, -31.7707) (175.1236, -31.7913) (175.2798, -31.8108) (175.4364, -31.8294) (175.5933, -31.847) (175.7505, -31.8637) (175.908, -31.8793) (176.0657, -31.8939) (176.2238, -31.9076) (176.3821, -31.9204) (176.5407, -31.9322) (176.6995, -31.9431) (176.8586, -31.9532) (177.0179, -31.9623) (177.1775, -31.9705) (177.3372, -31.9779) (177.4972, -31.9844) (177.6575, -31.99) (177.8179, -31.9948) (177.9785, -31.9987) (178.1394, -32.0017) (178.3004, -32.004) (178.4617, -32.0054) (178.6231, -32.006) (178.7847, -32.0057) (178.9465, -32.0047) (179.1085, -32.0028) (179.2706, -32.0002) (179.4329, -31.9967) (179.5954, -31.9925) (179.758, -31.9875) (179.9208, -31.9817) (180.0837, -31.9751) (180.2468, -31.9678) (180.41, -31.9597) (180.5733, -31.9508) (180.7368, -31.9412) (180.9005, -31.9308) (181.0642, -31.9197) (181.2281, -31.9078) (181.3921, -31.8952) (181.5563, -31.8819) (181.7205, -31.8678) (181.8848, -31.853) (182.0164, -31.8406) (182.1152, -31.8309) (182.181, -31.8243) (182.2139, -31.821) knots 0 0 0 0 0 0 0.01428571 0.02857143 0.04285714 0.05714286 0.07142857 0.08571429 0.1 0.11428571 0.12857143 0.14285714 0.15714286 0.17142857 0.18571429 0.2 0.21428571 0.22857143 0.24285714 0.25714286 0.27142857 0.28571429 0.3 0.31428571 0.32857143 0.34285714 0.35714286 0.37142857 0.38571429 0.4 0.41428571 0.42857143 0.44285714 0.45714286 0.47142857 0.48571429 0.5 0.51428571 0.52857143 0.54285714 0.55714286 0.57142857 0.58571429 0.6 0.61428571 0.62857143 0.64285714 0.65714286 0.67142857 0.68571429 0.7 0.71428571 0.72857143 0.74285714 0.75714286 0.77142857 0.78571429 0.8 0.81428571 0.82857143 0.84285714 0.85714286 0.87142857 0.88571429 0.9 0.91428571 0.92857143 0.94285714 0.95714286 0.97142857 0.98571429 1 1 1 1 1 1
  arc A143 (182.2139, -31.821) -> (183.8567, -27.855) centre (111, 0) ccw
  spline S71 degree 5 poles (183.8567, -27.855) (183.8358, -27.8294) (183.7939, -27.7782) (183.7309, -27.7015) (183.6466, -27.5997) (183.5409, -27.473) (183.4347, -27.3469) (183.3281, -27.2214) (183.221, -27.0965) (183.1135, -26.9723) (183.0056, -26.8486) (182.8972, -26.7256) (182.7884, -26.6031) (182.6792, -26.4814) (182.5695, -26.3602) (182.4594, -26.2397) (182.3488, -26.1199) (182.2378, -26.0007) (182.1264, -25.8821) (182.0145, -25.7642) (181.9021, -25.647) (181.7894, -25.5305) (181.6762, -25.4147) (181.5625, -25.2996) (181.4484, -25.1851) (181.3338, -25.0714) (181.2188, -24.9584) (181.1034, -24.8461) (180.9875, -24.7345) (180.8711, -24.6237) (180.7543, -24.5136) (180.637, -24.4043) (180.5193, -24.2957) (180.4011, -24.1879) (180.2825, -24.081) (180.1634, -23.9748) (180.0438, -23.8694) (179.9238, -23.7648) (179.8033, -23.661) (179.6823, -23.5581) (179.5608, -23.456) (179.4389, -23.3548) (179.3165, -23.2545) (179.1936, -23.1551) (179.0702, -23.0566) (178.9464, -22.959) (178.822, -22.8624) (178.6972, -22.7666) (178.5719, -22.6718) (178.446, -22.578) (178.3197, -22.4853) (178.1928, -22.3936) (178.0653, -22.3031) (177.9373, -22.2137) (177.8088, -22.1255) (177.6797, -22.0383) (177.5501, -21.9522) (177.4201, -21.8671) (177.2895, -21.7831) (177.1584, -21.7003) (177.0266, -21.619) (176.894, -21.5395) (176.7606, -21.4619) (176.6264, -21.3863) (176.4914, -21.3123) (176.356, -21.2395) (176.2202, -21.1677) (176.084, -21.0968) (175.9473, -21.0272) (175.8096, -20.9601) (175.6704, -20.897) (175.5573, -20.851) (175.4713, -20.8195) (175.4134, -20.8) (175.3843, -20.7906) knots -1 -1 -1 -1 -1 -1 -0.98571429 -0.97142857 -0.95714286 -0.94285714 -0.92857143 -0.91428571 -0.9 -0.88571429 -0.87142857 -0.85714286 -0.84285714 -0.82857143 -0.81428571 -0.8 -0.78571429 -0.77142857 -0.75714286 -0.74285714 -0.72857143 -0.71428571 -0.7 -0.68571429 -0.67142857 -0.65714286 -0.64285714 -0.62857143 -0.61428571 -0.6 -0.58571429 -0.57142857 -0.55714286 -0.54285714 -0.52857143 -0.51428571 -0.5 -0.48571429 -0.47142857 -0.45714286 -0.44285714 -0.42857143 -0.41428571 -0.4 -0.38571429 -0.37142857 -0.35714286 -0.34285714 -0.32857143 -0.31428571 -0.3 -0.28571429 -0.27142857 -0.25714286 -0.24285714 -0.22857143 -0.21428571 -0.2 -0.18571429 -0.17142857 -0.15714286 -0.14285714 -0.12857143 -0.11428571 -0.1 -0.08571429 -0.07142857 -0.05714286 -0.04285714 -0.02857143 -0.01428571 0 0 0 0 0 0
  line L71 (175.3843, -20.7906) -> (174.7851, -20.5971)
  arc A144 (173.4789, -18.1364) -> (174.7851, -20.5971) centre (175.3996, -18.6939) ccw
  circle A145 centre (111, 0) radius 2.5
sketch "Base Circle (2)" plane through (0, 0, 0) normal (0, 0, 1) x (1, 0, 0)
  circle A0 centre (0, 0) radius 29.058
  circle A1 centre (0, 0) radius 14.5
extrude "Extrude10" add sketch "Base Circle (2)" along normal blind 4 separate body makes body 6